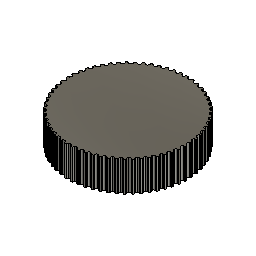
gear_63z (Autodesk Fusion 360 design; units mm, degrees)
Autodesk Fusion 360 part; units mm, degrees
sketch "Sketch1" plane through (0, 0, 0) normal (0, 0, 1) x (1, 0, 0) in component "gt2 pulley"
  circle A0 centre (0, 0) radius 20.0535 construction
  circle A1 centre (0, 0) radius 19.0495 construction
  line L0 (0, 0) -> (0, 20.0535) construction
  line L1 (0, 0) -> (0.9996, 20.0286) construction
  line L2 (0, 0) -> (1.406, 20.0042) construction
  circle A2 centre (0, 0) radius 19.7995 construction
  arc A3 (0.3922, 19.6614) -> (0.4646, 19.3673) centre (1.3882, 19.7508) ccw
  circle A4 centre (0, 0) radius 19.6495 construction
  arc A5 (0.2446, 19.798) -> (0, 19.7995) centre (0, 0) ccw
  arc A6 (0.3922, 19.6614) -> (0.2446, 19.798) centre (0.2428, 19.648) ccw
  arc A7 (0.4646, 19.3673) -> (0.9495, 19.0258) centre (0.9772, 19.5802) ccw
  arc A8 (0, 19.7995) -> (-0.2446, 19.798) centre (0, 0) ccw
  arc A9 (-0.2446, 19.798) -> (-0.3922, 19.6614) centre (-0.2428, 19.648) ccw
  arc A10 (-0.4646, 19.3673) -> (-0.3922, 19.6614) centre (-1.3882, 19.7508) ccw
  arc A11 (-0.9495, 19.0258) -> (-0.4646, 19.3673) centre (-0.9772, 19.5801) ccw
  arc A12 (0.9495, 19.0258) -> (-0.9495, 19.0258) centre (0, 0) ccw
  point P0 (1.3882, 19.7508)
  point P1 (0, 19.7995)
  dimension "d18" = 40.107
  dimension "d19" = 2.857
  dimension "d22" = 1.004
  dimension "d24" = 0.75
  dimension "d26" = 1
  dimension "d27" = 0.15
  dimension "d28" = 0.15
  dimension "d47" = 0.555
  dimension "d52" = 3.812
  constraint coincident A0.centre A1.centre
  constraint coincident A0 L0.end
  constraint vertical L0
  constraint coincident A0 L1.end
  constraint coincident A0 L2.end
  constraint concentric A1 A2
  constraint coincident A1 A7.end
  constraint coincident L1 A7.end
  constraint coincident A2 P0
  constraint coincident L2 P0
  constraint coincident P0 A3.centre
  constraint coincident A2 P1
  constraint coincident L0 P1
  constraint concentric A2 A4
  constraint coincident P1 A5.end
  constraint coincident A4 A6.centre
  constraint coincident A3.start A6.start
  constraint tangent A3 A6
  constraint tangent A3 A7
  constraint symmetric L0 A7.end A11.start
  constraint symmetric L0 A3.start A9.end
  constraint symmetric L0 A3.end A10.start
  constraint symmetric L0 A3 A10
  constraint symmetric L0 A5.start A8.end
  constraint symmetric L0 P1 A5.end
  constraint symmetric L0 A5 A8
  constraint symmetric L0 A6 A9
  constraint symmetric L0 A7 A11
  constraint coincident A1 A11.start
  constraint tangent A1 A7
  constraint coincident L1 A7.centre
  measures "d18" diameter of A0
  measures "d19" angle of L0 L1
  measures "d22" distance of A0 A1
  measures "d24" distance of A1 A2
  measures "d26" radius of A3
  measures "d27" distance of A2 A4
  measures "d28" radius of A6
  measures "d47" radius of A7
extrude "Extrude1" add sketch "Sketch1" along normal blind 10 makes body 1
pattern_circular "C-Pattern1" count 63 over 360 about axis through (0, 0, 1.75) along (0, 0, 1) of bodies 1 makes body 2 at (-2.0017, 18.9441, 6.6667) makes body 3 at (-3.0477, 18.8041, 3.3333) makes body 4 at (-6.3166, 17.9718, 6.6667) makes body 5 at (-8.0746, 17.2536, 6.6667) makes body 6 at (-8.455, 17.0704, 6.6667) makes body 7 at (-10.818, 15.6798, 6.6667) makes body 8 at (-11.6697, 15.0566, 3.3333) makes body 9 at (-13.1109, 13.8199, 3.3333) makes body 10 at (-14.4218, 12.4458, 3.3333) makes body 11 at (-16.3908, 9.707, 6.6667) makes body 12 at (-16.9995, 8.5965, 6.6667) makes body 13 at (-17.9187, 6.4657, 6.6667) makes body 14 at (-18.4734, 4.6494, 6.6667) makes body 15 at (-18.7782, 3.2039, 6.6667) makes body 16 at (-18.9268, 2.1591, 3.3333) makes body 17 at (-19.0477, 0.2639, 3.3333) makes body 18 at (-18.8883, -2.4734, 6.6667) makes body 19 at (-18.5481, -4.3418, 6.6667) makes body 20 at (-18.0909, -5.9669, 6.6667) makes body 21 at (-17.6545, -7.1556, 3.3333) makes body 22 at (-16.1156, -10.1573, 6.6667) makes body 23 at (-15.8866, -10.5119, 3.3333) makes body 24 at (-14.2129, -12.6837, 6.6667) makes body 25 at (-13.4887, -13.4514, 3.3333) makes body 26 at (-11.4179, -15.2485, 6.6667) makes body 27 at (-10.5559, -15.8574, 3.3333) makes body 28 at (-8.9246, -16.8296, 6.6667) makes body 29 at (-5.8163, -18.1399, 6.6667) makes body 30 at (-4.5983, -18.4862, 6.6667) makes body 31 at (-3.5675, -18.7125, 3.3333) makes body 32 at (-0.2111, -19.0484, 6.6667) makes body 33 at (0.2111, -19.0484, 3.3333) makes body 34 at (2.9435, -18.8207, 6.6667) makes body 35 at (5.2102, -18.3232, 6.6667) makes body 36 at (6.6144, -17.8643, 6.6667) makes body 37 at (8.1701, -17.2086, 6.6667) makes body 38 at (10.023, -16.1995, 6.6667) makes body 39 at (11.5861, -15.121, 6.6667) makes body 40 at (12.4058, -14.4562, 3.3333) makes body 41 at (13.7835, -13.1491, 3.3333) makes body 42 at (15.5284, -11.0342, 6.6667) makes body 43 at (16.8543, -8.8779, 6.6667) makes body 44 at (17.0469, -8.5022, 3.3333) makes body 45 at (17.8087, -6.7626, 3.3333) makes body 46 at (18.3936, -4.9559, 3.3333) makes body 47 at (18.9145, -2.2639, 6.6667) makes body 48 at (19.0109, -1.213, 3.3333) makes body 49 at (18.9881, 1.5288, 6.6667) makes body 50 at (18.8743, 2.578, 3.3333) makes body 51 at (18.1876, 5.6654, 6.6667) makes body 52 at (17.6939, 7.0577, 6.6667) makes body 53 at (16.9032, 8.7844, 6.6667) makes body 54 at (16.3908, 9.707, 3.3333) makes body 55 at (14.8275, 11.9595, 6.6667) makes body 56 at (13.563, 13.3764, 6.6667) makes body 57 at (11.6697, 15.0566, 6.6667) makes body 58 at (11.3332, 15.3115, 3.3333) makes body 59 at (8.455, 17.0704, 6.6667) makes body 60 at (7.3021, 17.5944, 6.6667) makes body 61 at (4.9049, 18.4072, 6.6667) makes body 62 at (4.4958, 18.5114, 3.3333) makes body 63 at (2.6303, 18.8671, 3.3333)
sketch "Sketch2" plane through (0, 0, 10) normal (0, 0, 1) x (-1, 0, 0)
  arc A0 (-7.9986, -17.9652) -> (-7.9156, -18.1484) centre (-7.8557, -18.0109) ccw
  arc A1 (-7.9156, -18.1484) -> (-7.4649, -18.3384) centre (0, 0) ccw
  arc A2 (-7.4649, -18.3384) -> (-7.2758, -18.2699) centre (-7.4083, -18.1995) ccw
  arc A3 (-7.0948, -18.027) -> (-7.2758, -18.2699) centre (-6.3927, -18.7391) ccw
  arc A4 (-6.5153, -17.9007) -> (-7.0948, -18.027) centre (-6.7051, -18.4222) ccw
  arc A5 (-8.2653, -17.163) -> (-6.5153, -17.9007) centre (0, 0) ccw
  arc A6 (-7.9511, -17.666) -> (-8.2653, -17.163) centre (-8.5061, -17.6631) ccw
  arc A7 (-7.9986, -17.9652) -> (-7.9511, -17.666) centre (-8.9511, -17.6607) ccw
  circle A8 centre (0, 0) radius 19.0495
  constraint coincident A1.centre A5.centre
extrude "Extrude2" add sketch "Sketch2" against normal blind 10 contours A5 A8 bodies 1 2 3 4 5 6 7 8 9 10 11 12 13 14 15 16 17 18 19 20 21 22 23 24 25 26 27 28 29 30 31 32 33 34 35 36 37 38 39 40 41 42 43 44 45 46 47 48 49 50 51 52 53 54 55 56 57 58 59 60 61 62 63
extrude "Extrude4" [suppressed] in component "gt2 pulley"
pattern_circular "C-Pattern7" [suppressed] in component "gt2 pulley"
extrude "Extrude3" [suppressed] in component "gt2 pulley"
pattern_circular "C-Pattern6" [suppressed] in component "gt2 pulley"
extrude "Extrude2'" [suppressed] in component "gt2 pulley"
pattern_circular "C-Pattern5" [suppressed] in component "gt2 pulley"
extrude "Extrude1'" [suppressed] in component "gt2 pulley"
pattern_circular "C-Pattern4" [suppressed] in component "gt2 pulley"
pattern_circular "C-Pattern3" [suppressed] in component "gt2 pulley"
pattern_circular "C-Pattern2" [suppressed] in component "gt2 pulley"
pattern_circular "C-Pattern1'" [suppressed] in component "gt2 pulley"
copy_body "Body->Comp1" [suppressed] in component "Component"
copy_body "Body->Comp2" [suppressed] in component "Component'"
copy_body "Body->Comp3" [suppressed] in component "Component''"
copy_body "Body->Comp4" [suppressed] in component "Component'''"
copy_body "Body->Comp5" [suppressed] in component "Component''''"
copy_body "Body->Comp6" [suppressed] in component "Component'''''"
copy_body "Body->Comp7" [suppressed] in component "Component''''''"
copy_body "Body->Comp8" [suppressed] in component "Component'''''''"
copy_body "Body->Comp9" [suppressed] in component "Component''''''''"
copy_body "Body->Comp10" [suppressed] in component "Component'''''''''"
copy_body "Body->Comp11" [suppressed] in component "Component''''''''''"
copy_body "Body->Comp12" [suppressed] in component "Component'''''''''''"
copy_body "Body->Comp13" [suppressed] in component "Component''''''''''''"
copy_body "Body->Comp14" [suppressed] in component "Component'''''''''''''"
copy_body "Body->Comp15" [suppressed] in component "Component''''''''''''''"
copy_body "Body->Comp16" [suppressed] in component "Component'''''''''''''''"
copy_body "Body->Comp17" [suppressed] in component "Component''''''''''''''''"
copy_body "Body->Comp18" [suppressed] in component "Component'''''''''''''''''"
copy_body "Body->Comp19" [suppressed] in component "Component''''''''''''''''''"
copy_body "Body->Comp20" [suppressed] in component "Component'''''''''''''''''''"
component "gt2 pulley" placed x (1, 0, 0) y (0, 1, 0) z (0, 0, 1) at (0, 0, 0)
equation "NumTeeth = 63" comment "min 20"
equation "ToothPitch = 2 mm"
equation "PullyDia = NumTeeth * ToothPitch / PI"
equation "ToothAng = ( ( 360 / NumTeeth ) * 1 deg )"
equation "TransOffsetAngle = ToothAng * 0.2"
equation "Sholulder_Radius = 0.15 mm"
equation "Root_Radius = 0.555 mm"
equation "TransRadius = 1 mm"
equation "ToolHeight = 0.75 mm"
equation "PLD = 0.254 mm"
equation "d18 = PullyDia"
equation "d19 = ToothAng / 2"
equation "d22 = PLD + ToolHeight"
equation "d24 = ToolHeight"
equation "d26 = TransRadius"
equation "d27 = Sholulder_Radius"
equation "d31 = NumTeeth"
equation "d33 = NumTeeth"
equation "d35 = NumTeeth"
equation "d37 = NumTeeth"
equation "d41 = NumTeeth"
equation "d45 = NumTeeth"
equation "d47 = Root_Radius"
equation "d50 = NumTeeth"
